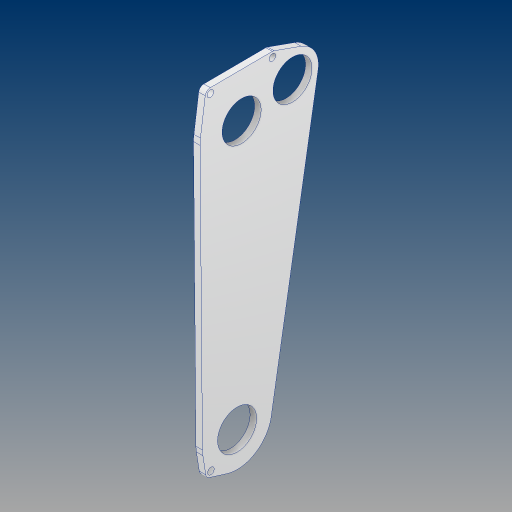
# Autodesk Inventor part: INTK_001_PulleyCover2
Saved by Autodesk Inventor 2024.3 (Build 283343000, 343)
## iProperties
Created: 2024-08-03
Part Number: INTK_001_PulleyCover2
Material: Aluminum 6061
Document SubType Name: Modeling
Designer: Kenji
Density: 2.7 g/cm^3
Appearance: Aluminum - Flat
Author: Kenji
Autodesk Inventor part; units mm, degrees
ref_plane "YZ Plane" through (0, 0, 0) normal (1, 0, 0) x (0, 1, 0)
ref_plane "XZ Plane" through (0, 0, 0) normal (0, 1, 0) x (-1, 0, 0)
ref_plane "XY Plane" through (0, 0, 0) normal (0, 0, 1) x (1, 0, 0)
sketch "Sketch1" plane through (0, 0, 0) normal (1, 0, 0) x (0, 1, 0)
  circle A0 centre (0, 0) radius 25.4 construction
  line L0 (0, 0) -> (0, -40.6423) construction
  line L1 (0, -40.6423) -> (202.0601, -40.6423) construction
  circle A1 centre (202.0601, -40.6423) radius 19.05 construction
  line L2 (202.0601, -40.6423) -> (194.4086, -40.6423) construction
  line L3 (194.4086, -40.6423) -> (194.4086, -3.3186) construction
  circle A2 centre (194.4086, -3.3186) radius 30.48 construction
  line L4 (16.6237, -19.2045) -> (-16.6237, 19.2045) construction
  circle A3 centre (-16.6237, 19.2045) radius 2.3876
  circle A4 centre (-16.6237, 19.2045) radius 3.81 construction
  line L5 (218.2698, 15.6466) -> (220.2582, 17.227) construction
  line L6 (218.497, -21.9942) -> (220.5043, -23.5505) construction
  line L7 (194.4086, -3.3186) -> (194.4086, 27.1614) construction
  circle A5 centre (223.5154, -25.885) radius 2.3876
  circle A6 centre (223.2408, 19.5976) radius 2.3876
  circle A7 centre (223.2408, 19.5976) radius 3.81 construction
  circle A8 centre (223.5154, -25.885) radius 3.81 construction
  line L8 (227.0508, 19.6206) -> (227.3253, -25.862)
  line L9 (227.1033, -27.1668) -> (219.9997, -47.0511)
  line L10 (198.8808, -59.4252) -> (-4.2391, -25.0438)
  arc A9 (227.1033, -27.1668) -> (227.3253, -25.862) centre (223.5154, -25.885) ccw
  arc A10 (198.8808, -59.4252) -> (219.9997, -47.0511) centre (202.0601, -40.6423) ccw
  line L11 (-4.0136, 25.0809) -> (-17.2257, 22.9666)
  line L12 (-20.2607, 20.3395) -> (-24.2467, 7.5667)
  arc A11 (-0.2302, 25.399) -> (-4.0136, 25.0809) centre (0, 0) ccw
  arc A12 (-17.2257, 22.9666) -> (-20.2607, 20.3395) centre (-16.6237, 19.2045) ccw
  arc A13 (-24.2467, 7.5667) -> (-4.2391, -25.0438) centre (0, 0) ccw
  arc A14 (227.0508, 19.6206) -> (223.7658, 23.3713) centre (223.2408, 19.5976) ccw
  circle A15 centre (194.4086, -3.3186) radius 14.2875
  circle A16 centre (202.0601, -40.6423) radius 14.2875
  circle A17 centre (0, 0) radius 14.2875
  line L13 (-0.2302, 25.399) -> (194.1324, 27.1602)
  line L14 (223.7658, 23.3713) -> (198.608, 26.8708)
  arc A18 (198.608, 26.8708) -> (194.1324, 27.1602) centre (194.4086, -3.3186) ccw
  dimension "d0" = 50.8
  dimension "d1" = 40.6423
  dimension "d2" = 202.0601
  dimension "d3" = 38.1
  dimension "d4" = 7.6515
  dimension "d5" = 37.3238
  dimension "d6" = 60.96
  dimension "d7" = 40.88
  dimension "d8" = 4.7752
  dimension "d9" = 7.62
  dimension "d10" = 2.54
  dimension "d11" = 2.54
  dimension "d12" = 51.522
  dimension "d13" = 127.786
  dimension "d14" = 4.7752
  dimension "d15" = 4.7752
  dimension "d16" = 7.62
  dimension "d17" = 7.62
  dimension "d18" = 28.575
  dimension "d19" = 28.575
  dimension "d20" = 28.575
  constraints: 35 point on circle, 30 end point, 19 centre point, 15 tangent, 10 coincident, 7 concentric, 5 point on line, 1 collinear, 1 horizontal, 1 midpoint, 1 perpendicular, 1 vertical
  measures "d0" diameter of A0
  measures "d1" distance of L0.start L0.end
  measures "d2" distance of L0.end L1.end
  measures "d3" diameter of A1
  measures "d4" distance of L2.start L2.end
  measures "d5" distance of L2.end L3.end
  measures "d6" diameter of A2
  measures "d7" angle of L4 L0
  measures "d8" diameter of A3
  measures "d9" diameter of A4
  measures "d10" distance of L5.start L5.end
  measures "d11" distance of L6.start L6.end
  measures "d12" angle of L7 L5
  measures "d13" angle of L6 L7
  measures "d14" diameter of A5
  measures "d15" diameter of A6
  measures "d16" diameter of A7
  measures "d17" diameter of A8
  measures "d18" diameter of A15
  measures "d19" diameter of A16
  measures "d20" diameter of A17
extrude "Extrusion2" add sketch "Sketch1" along normal blind 4.7625
body "Solid2"
